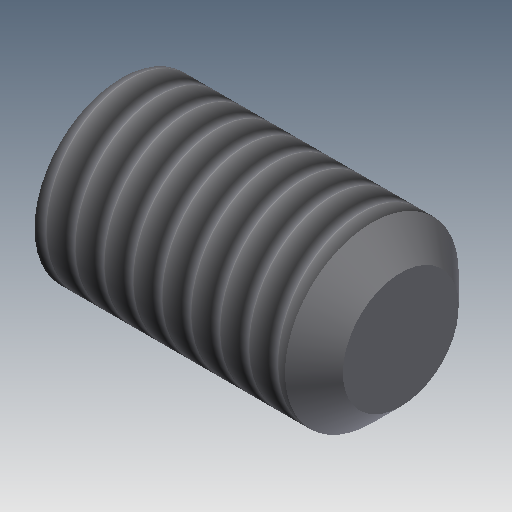
# Autodesk Inventor part: Hexagon socket set screw with flat point DIN 913 - M3x5
Saved by Autodesk Inventor 2019.4 (Build 234330000, 330)
## iProperties
Category: PARTsolutions
Company: MISUMI
Created: 2019-06-16
Part Number: Hexagon socket set screw with flat point DIN 913 - M3x5
Material: 一般
Catalog Web Link: www.cadenas.de
Description: DIN 913-Hexagon socket set screw with flat point
Vendor: MISUMI
Document SubType Name: Modeling
Designer: psadmin
Manufacturer: MISUMI
Mass: 0.0301497 g
Surface Area: 0.671354 cm^2
Volume: 0.0301497 cm^3
Density: 1 g/cm^3
Appearance: PSOLRGB-192-192-192
PSOL_IDENT_0: {$CADENAS_DATA\23d-libs\misumi\metric\accessories\din_913.prj},254 {VTYP=3D},{NB=Hexagon socket set
PSOL_IDENT_1: screw with flat point DIN 913 - M3x5},{LINA=Hexagon socket set screw with flat point DIN 913 - M3x5}
PSOL_IDENT_2: ,{NN=DIN 913},{DATE=17.06.2016 05:56:50},{GEOMDATE=17.02.2014 00:00:00},{VERSION=v1},{LINEID=250},{W
PSOL_IDENT_3: BVAR=},{WBNUMERIC=}  {NB=Gewindestift DIN 913 - M3x5},{LINA=Gewindestift DIN 913 - M3x5},{KT=X},{IDN
PSOL_IDENT_4: R=},{NENN=M3x5},{D=3.000},{D3=2.387},{P=0.500},{L=5.000},{DP=2.000},{S=1.500},{T=2.000}
NN: DIN 913
NT: Hexagon socket set screw with flat point
NB: Headless pin DIN 913 - M3x5
NBSYN: Headless pin DIN 913 - $NENN.
LINA: Headless pin DIN 913 - M3x5
ROWDESC: M3x5
D: 3
D3: 2.387
P: 0.5
L: 5
DP: 2
S: 1.5
T: 2
SUPPLIER: MISUMI
ARTICLENO: Hexagon socket set screw with flat point DIN 913 - M3x5
BOMINFO: Hexagon socket set screw with flat point DIN 913 - M3x5
CREATOR: CADENAS GmbH
Title: Hexagon socket set screw with flat point DIN 913 - M3x5
Author: Cadenas PARTsolutions
Comments: Hexagon socket set screw with flat point
Autodesk Inventor part; units mm, degrees
sketch "Sketch_1" plane through (0, 0, 0) normal (0, 0, 1) x (1, 0, 0)
  line L0 (0.5, 0) -> (5, 0)
  line L1 (5, 0) -> (5, -1)
  line L2 (5, -1) -> (4.5, -1.5)
  line L3 (4.5, -1.5) -> (0.177, -1.5)
  line L4 (0.177, -1.5) -> (0, -1.1935)
  line L5 (0, -1.1935) -> (0, -0.866)
  line L6 (0, -0.866) -> (0.5, 0)
  line L7 (0.5, 0) -> (5, 0)
  constraints: 16 end point
revolve "Revolution1" add sketch "Sketch_1" angle 360 about axis through (0.5, 0, 0) along (1, 0, 0)
thread "Thread1" size "M3x0.5" class "6g" standard "ISO Metric profile" full length
sketch "Sketch_2" plane through (0, 0, 0) normal (1, 0, 0) x (0, 1, 0)
  line L0 (0, 0.866) -> (-0.75, 0.433)
  line L1 (-0.75, 0.433) -> (-0.75, -0.433)
  line L2 (-0.75, -0.433) -> (0, -0.866)
  line L3 (0, -0.866) -> (0.75, -0.433)
  line L4 (0.75, -0.433) -> (0.75, 0.433)
  line L5 (0.75, 0.433) -> (0, 0.866)
  constraints: 12 end point
extrude "Extrusion1" cut sketch "Sketch_2" along normal blind 2
ref_plane "IP1_XY" through (0, 0, 0) normal (1, 0, 0) x (0, 0, -1)
ref_plane "IP1_YZ" through (0, 0, 0) normal (0, 0, -1) x (0, 1, 0)
ref_plane "IP1_ZX" through (0, 0, 0) normal (0, 1, 0) x (1, 0, 0)
ref_plane "IP2_XY" through (5, 0, 0) normal (1, 0, 0) x (0, 0, -1)
ref_plane "IP2_YZ" through (5, 0, 0) normal (0, 0, -1) x (0, 1, 0)
ref_plane "IP2_ZX" through (5, 0, 0) normal (0, 1, 0) x (1, 0, 0)
body "Solid1"
